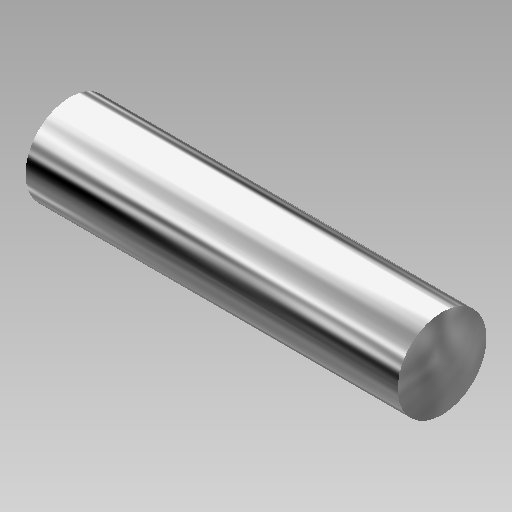
# Autodesk Inventor part: pin
Saved by Autodesk Inventor 2018.1 (Build 221171000, 171)
## iProperties
Created: 2013-08-27
Part Number: pin
Material: Generic
Document SubType Name: Modeling
Designer: Konstantin
Density: 1 g/cm^3
Appearance: Default
Mass: 0.0899405 g
Surface Area: 1.3258 cm^2
Volume: 0.0899405 cm^3
Author: Konstantin
Autodesk Inventor part; units mm, degrees
ref_plane "YZ Plane" through (0, 0, 0) normal (1, 0, 0) x (0, 1, 0)
ref_plane "XZ Plane" through (0, 0, 0) normal (0, 1, 0) x (-1, 0, 0)
ref_plane "XY Plane" through (0, 0, 0) normal (0, 0, 1) x (1, 0, 0)
sketch "Sketch1" plane through (0, 0, 0) normal (0, 0, 1) x (1, 0, 0)
  line L0 (0, 0) -> (12.9, 0)
  line L1 (12.7232, 1.5) -> (0.1768, 1.5)
  arc A0 (12.9, 0) -> (12.7232, 1.5) centre (6.45, 0) ccw
  arc A1 (0.1768, 1.5) -> (0, 0) centre (6.45, 0) ccw
  constraints: 4 end point, 4 point on circle, 2 centre point, 2 horizontal, 1 midpoint, 1 parallel, 1 other
revolve "Revolution1" add sketch "Sketch1" angle 360 about axis through (0, 0, 0) along (1, 0, 0)
body "Solid1"
